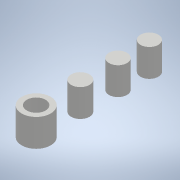
# Autodesk Inventor part: Тест
Saved by Autodesk Inventor 2020 (Build 240168000, 168)
## iProperties
Created: 2021-05-01
Part Number: Тест
Material: Типовые
Document SubType Name: ЛистМат
Designer: I_Love_U_Bogdan
Density: 1 g/cm^3
Appearance: По умолчанию
Sheet Metal Rule: По умолчанию
Author: I_Love_U_Bogdan
Autodesk Inventor part; units mm, degrees
ref_plane "YZ Plane" through (0, 0, 0) normal (1, 0, 0) x (0, 1, 0)
ref_plane "XZ Plane" through (0, 0, 0) normal (0, 1, 0) x (-1, 0, 0)
ref_plane "XY Plane" through (0, 0, 0) normal (0, 0, 1) x (1, 0, 0)
sketch "Эскиз1" plane through (0, 0, 0) normal (0, 1, 0) x (-1, 0, 0)
  circle A0 centre (0, 0) radius 5.1
  circle A1 centre (0, 0) radius 7.9
  circle A2 centre (0, -23.9962) radius 5
  circle A3 centre (0, -44.4623) radius 4.9
  circle A4 centre (0, -61.5505) radius 4.85
  dimension "d0" = 10.2
  dimension "d1" = 15.8
  dimension "d2" = 10
  dimension "d3" = 9.8
  dimension "d4" = 9.7
  constraints: 5 centre point, 2 coincident
  measures "d0" diameter of A0
  measures "d1" diameter of A1
  measures "d2" diameter of A2
  measures "d3" diameter of A3
  measures "d4" diameter of A4
extrude "Выдавливание1" add sketch "Эскиз1" along normal blind 15
sketch "Эскиз2" plane through (0, 15, -23.9962) normal (0, 1, 0) x (1, 0, 0)
  line L0 (-2.1701, 1.6946) -> (2.4044, 1.6946) construction
  line L1 (2.4044, 1.6946) -> (2.4044, -1.4794) construction
  line L2 (2.4044, -1.4794) -> (-2.1701, -1.4794) construction
  line L3 (-2.1701, -1.4794) -> (-2.1701, 1.6946) construction
  line L4 (-3.1832, 22.0453) -> (2.6609, 22.0453) construction
  line L5 (2.6609, 22.0453) -> (2.6609, 18.1698) construction
  line L6 (2.6609, 18.1698) -> (-3.1832, 18.1698) construction
  line L7 (-3.1832, 18.1698) -> (-3.1832, 22.0453) construction
  line L8 (-2.9124, 39.0147) -> (2.9316, 39.0147) construction
  line L9 (2.9316, 39.0147) -> (2.9316, 35.1466) construction
  line L10 (2.9316, 35.1466) -> (-2.9124, 35.1466) construction
  line L11 (-2.9124, 35.1466) -> (-2.9124, 39.0147) construction
  point P0 (0, -23.9962)
  constraints: 6 other
equation "\"Радиус_гибки\" = Толщина"
equation "\"Ширина_просечки\" = Толщина"
equation "\"Глубина_просечки\" = 0.5 * Толщина"
equation "\"Размер_просечки\" = 4 * Толщина"
equation "\"Мин_остаток\" = 2 * Толщина"
equation "\"Радиус_перехода\" = Радиус_гибки"
equation "\"Радиус_Якоби\" = Толщина"
equation "\"Размер_зазора\" = Толщина"
equation "\"Толщина\" = 0.5"
